Autodesk Fusion 360 part; units mm, degrees
(part 4 of 4)
sketch "Skizze66" plane through (0, 21.5, 0) normal (0, -1, 0) x (1, 0, 0)
  line L0 (56.5, -5) -> (51.5, -5)
  line L1 (51.5, -5) -> (51.5, -9.5)
  line L2 (51.5, -9.5) -> (31, -9.5)
  line L3 (31, -9.5) -> (31, -19.2)
  line L4 (31, -19.2) -> (32.5, -19.2)
  line L5 (32.5, -19.2) -> (32.5, -19)
  arc A0 (33.5, -18) -> (32.5, -19) centre (33.5, -19) ccw
  line L6 (33.5, -18) -> (38.5, -18)
  arc A1 (38.5, -18) -> (39.5, -17) centre (38.5, -17) ccw
  line L7 (39.5, -17) -> (39.5, -12)
  arc A2 (40.5, -11) -> (39.5, -12) centre (40.5, -12) ccw
  line L8 (40.5, -11) -> (56.5, -11)
  line L9 (56.5, -11) -> (56.5, -5)
  circle A3 centre (36, -14.5) radius 1.9
  line L10 (56.5, 5) -> (56.5, -5)
  line L11 (56.5, 5) -> (51.5, 5)
  line L12 (51.5, -5) -> (51.5, 5)
  line L13 (51.5, -5) -> (56.5, -5)
  circle A4 centre (-3.5, 16) radius 6.5
  line L14 (-21.5, -1.5) -> (-21.5, -23.5)
  line L15 (-21.5, -23.5) -> (5.5, -23.5)
  line L16 (5.5, -23.5) -> (5.5, -1.5)
  line L17 (5.5, -1.5) -> (-21.5, -1.5)
  line L18 (37.3325, 4.5) -> (48.5, 4.5)
  arc A5 (48.5, 4.5) -> (48.5, 7.5) centre (48.5, 6) ccw
  line L19 (48.5, 7.5) -> (37.3325, 7.5)
  arc A6 (37.3325, 7.5) -> (37.3325, 4.5) centre (37.3325, 6) ccw
  line L20 (12.5, 2.5057) -> (20.5, 2.5057)
  arc A7 (20.5, 2.5057) -> (20.5, 4.5057) centre (20.5, 3.5057) ccw
  line L21 (20.5, 4.5057) -> (12.5, 4.5057)
  arc A8 (12.5, 4.5057) -> (12.5, 2.5057) centre (12.5, 3.5057) ccw
  line L22 (12.5, -15.2086) -> (20.5, -15.2086)
  arc A9 (20.5, -15.2086) -> (20.5, -13.2086) centre (20.5, -14.2086) ccw
  line L23 (20.5, -13.2086) -> (12.5, -13.2086)
  arc A10 (12.5, -13.2086) -> (12.5, -15.2086) centre (12.5, -14.2086) ccw
  arc A11 (-34, 4.5) -> (-34, 7.5) centre (-34, 6) ccw
  line L24 (-34, 7.5) -> (-45, 7.5)
  arc A12 (-45, 7.5) -> (-45, 4.5) centre (-45, 6) ccw
  line L25 (-45, 4.5) -> (-34, 4.5)
  arc A13 (-34, -13.5) -> (-34, -10.5) centre (-34, -12) ccw
  line L26 (-34, -10.5) -> (-45, -10.5)
  arc A14 (-45, -10.5) -> (-45, -13.5) centre (-45, -12) ccw
  line L27 (-45, -13.5) -> (-34, -13.5)
  arc A15 (-34, 10.5) -> (-34, 13.5) centre (-34, 12) ccw
  line L28 (-34, 13.5) -> (-45, 13.5)
  arc A16 (-45, 13.5) -> (-45, 10.5) centre (-45, 12) ccw
  line L29 (-45, 10.5) -> (-34, 10.5)
  line L30 (12.5, -10.78) -> (20.5, -10.78)
  arc A17 (20.5, -10.78) -> (20.5, -8.78) centre (20.5, -9.78) ccw
  line L31 (20.5, -8.78) -> (12.5, -8.78)
  arc A18 (12.5, -8.78) -> (12.5, -10.78) centre (12.5, -9.78) ccw
  line L32 (20.5, 8.9343) -> (12.5, 8.9343)
  arc A19 (12.5, 8.9343) -> (12.5, 6.9343) centre (12.5, 7.9343) ccw
  line L33 (12.5, 6.9343) -> (20.5, 6.9343)
  arc A20 (20.5, 6.9343) -> (20.5, 8.9343) centre (20.5, 7.9343) ccw
  line L34 (37.3325, -1.5) -> (48.5, -1.5)
  arc A21 (48.5, -1.5) -> (48.5, 1.5) centre (48.5, 0) ccw
  line L35 (48.5, 1.5) -> (37.3325, 1.5)
  arc A22 (37.3325, 1.5) -> (37.3325, -1.5) centre (37.3325, 0) ccw
  arc A23 (20.5, -1.9228) -> (20.8852, 0) centre (20.5, -0.9228) ccw
  line L36 (20.8852, 0) -> (12.1148, 0)
  arc A24 (12.1148, 0) -> (12.5, -1.9228) centre (12.5, -0.9228) ccw
  line L37 (12.5, -1.9228) -> (20.5, -1.9228)
  line L38 (20.5, -22.0657) -> (20.5, -19.6371)
  arc A25 (20.5, -19.6371) -> (20.5, -17.6371) centre (20.5, -18.6371) ccw
  line L39 (20.5, -17.6371) -> (12.5, -17.6371)
  arc A26 (12.5, -17.6371) -> (12.5, -19.6371) centre (12.5, -18.6371) ccw
  line L40 (12.5, -19.6371) -> (12.5, -22.0657)
  arc A27 (12.5, -22.0657) -> (12.5, -24.0657) centre (12.5, -23.0657) ccw
  line L41 (12.5, -24.0657) -> (20.5, -24.0657)
  arc A28 (20.5, -24.0657) -> (20.5, -22.0657) centre (20.5, -23.0657) ccw
  line L42 (-34, 1.5) -> (-45, 1.5)
  arc A29 (-45, 1.5) -> (-45, -1.5) centre (-45, 0) ccw
  line L43 (-45, -1.5) -> (-34, -1.5)
  arc A30 (-34, -1.5) -> (-34, 1.5) centre (-34, 0) ccw
  arc A31 (-34, -7.5) -> (-34, -4.5) centre (-34, -6) ccw
  line L44 (-34, -4.5) -> (-45, -4.5)
  arc A32 (-45, -4.5) -> (-45, -7.5) centre (-45, -6) ccw
  line L45 (-45, -7.5) -> (-34, -7.5)
  line L46 (37.3325, -7.5) -> (48.5, -7.5)
  arc A33 (48.5, -7.5) -> (48.5, -4.5) centre (48.5, -6) ccw
  line L47 (48.5, -4.5) -> (37.3325, -4.5)
  arc A34 (37.3325, -4.5) -> (37.3325, -7.5) centre (37.3325, -6) ccw
  line L48 (-22.3, -10.5) -> (-30, -10.5)
  line L49 (-30, -10.5) -> (-30, -18.5)
  line L50 (-30, -18.5) -> (-22.3, -18.5)
  line L51 (-22.3, -18.5) -> (-22.3, -10.5)
  line L52 (36, 11) -> (56.5, 11)
  line L53 (56.5, 11) -> (56.5, -11)
  line L54 (56.5, -11) -> (36, -11)
  arc A35 (36, -11) -> (32.5, -14.5) centre (36, -14.5) ccw
  line L55 (32.5, -14.5) -> (32.5, -27.5)
  line L56 (32.5, -27.5) -> (-32, -27.5)
  line L57 (-32, -27.5) -> (-32, -25)
  arc A36 (-32, -25) -> (-36, -21) centre (-36, -25) ccw
  line L58 (-36, -21) -> (-43, -21)
  line L59 (-43, -21) -> (-57.5, -6.5)
  line L60 (-57.5, -6.5) -> (-57.5, 6.5)
  line L61 (-57.5, 6.5) -> (-43, 21)
  line L62 (-43, 21) -> (-36, 21)
  arc A37 (-36, 21) -> (-32, 25) centre (-36, 25) ccw
  line L63 (-32, 25) -> (-32, 27.5)
  line L64 (-32, 27.5) -> (10.5, 27.5)
  line L65 (10.5, 27.5) -> (10.5, 21.5)
  line L66 (10.5, 21.5) -> (12, 21.5)
  line L67 (12, 21.5) -> (12, 11.5)
  line L68 (12, 11.5) -> (21, 11.5)
  line L69 (21, 11.5) -> (21, 21.5)
  line L70 (21, 21.5) -> (22.5, 21.5)
  line L71 (22.5, 21.5) -> (22.5, 27.5)
  line L72 (22.5, 27.5) -> (32.5, 27.5)
  line L73 (32.5, 27.5) -> (32.5, 14.5)
  arc A38 (32.5, 14.5) -> (36, 11) centre (36, 14.5) ccw
  line L74 (20.5, -7.58) -> (20.5, -6.3514)
  arc A39 (20.5, -6.3514) -> (20.5, -4.3514) centre (20.5, -5.3514) ccw
  line L75 (20.5, -4.3514) -> (12.5, -4.3514)
  arc A40 (12.5, -4.3514) -> (12.5, -6.3514) centre (12.5, -5.3514) ccw
  line L76 (12.5, -6.3514) -> (12.5, -7.58)
  line L77 (12.5, -7.58) -> (20.5, -7.58)
  line L78 (51.5, 5) -> (56.5, 5)
  line L79 (56.5, 5) -> (56.5, 11)
  line L80 (56.5, 11) -> (40.5, 11)
  arc A41 (39.5, 12) -> (40.5, 11) centre (40.5, 12) ccw
  line L81 (39.5, 12) -> (39.5, 17)
  arc A42 (39.5, 17) -> (38.5, 18) centre (38.5, 17) ccw
  line L82 (38.5, 18) -> (33.5, 18)
  arc A43 (32.5, 19) -> (33.5, 18) centre (33.5, 19) ccw
  line L83 (32.5, 19) -> (32.5, 19.2)
  line L84 (32.5, 19.2) -> (31, 19.2)
  line L85 (31, 19.2) -> (31, 9.5)
  line L86 (31, 9.5) -> (51.5, 9.5)
  line L87 (51.5, 9.5) -> (51.5, 5)
  circle A44 centre (36, 14.5) radius 1.9
extrude "Extrusion72" cut sketch "Skizze66" against normal blind 3 contours L0 L1 L2 L3 L4 L5 L8 L9 L13 L53 L54 A35 L55 | L0 L10 L11 L12 L13 L53 L78 | L11 L52 L53 L73 A38 L78 L79 L80 L83 L84 L85 L86 L87 | A0 L6 A1 L7 A2 L54 A35 L55 | L52 L73 A38 A41 L81 A42 L82 A43 bodies 2
sketch "Skizze67" plane through (0, 16, 0) normal (0, -1, 0) x (1, 0, 0)
  circle A0 centre (-36, -25) radius 1.9
  line L0 (-18.0278, -27.5) -> (-18.0278, -26)
  line L1 (-18.0278, -26) -> (-23, -26)
  line L2 (-23, -26) -> (-31, -26)
  line L3 (-31, -26) -> (-31, -20)
  line L4 (-31, -20) -> (-41.8787, -20)
  line L5 (-41.8787, -20) -> (-51.5218, -10.3569)
  line L6 (-51.5218, -10.3569) -> (-51.5218, -5)
  line L7 (-51.5218, -5) -> (-57.5, -5)
  line L8 (-57.5, -5) -> (-57.5, -6.5)
  line L9 (-57.5, -6.5) -> (-42.5, -21.5)
  line L10 (-42.5, -21.5) -> (-38.922, -26.9266)
  arc A1 (-38.922, -26.9266) -> (-34.8649, -28.3108) centre (-36, -25) ccw
  line L11 (-34.8649, -28.3108) -> (-32.5, -27.5)
  line L12 (-32.5, -27.5) -> (-18.0278, -27.5)
  line L13 (-51.5218, 5) -> (-51.5218, -5)
  line L14 (-51.5218, 5) -> (-57.5, 5)
  line L15 (-57.5, -5) -> (-57.5, 5)
  line L16 (-57.5, -5) -> (-51.5218, -5)
  line L17 (-44.7071, 17.1716) -> (-47.5355, 14.3431)
  line L18 (-44.7071, 17.1716) -> (-45.7678, 18.2322)
  line L19 (-48.5962, 15.4038) -> (-45.7678, 18.2322)
  line L20 (-48.5962, 15.4038) -> (-47.5355, 14.3431)
extrude "Extrusion73" cut sketch "Skizze67" 3 faces at (-53.5145, 16, 7.2856) (-36.3402, 16, 21.0351) (24.5093, 16, -27) against normal blind 3 on bodies 2 bodies 2
extrude "Extrusion74" add 2 faces at (54.8333, 21.5, 8.5) (54.8333, 21.5, -8.5) along direction (0, 1, 0) blind 3 on bodies 1 bodies 1
extrude "Extrusion75" add 3 faces at (27.1759, 16, -27) (-53.5145, 16, 7.2856) (-53.5145, 16, -7.2856) along direction (0, 1, 0) blind 3 on bodies 1 bodies 1
sketch "Skizze68" plane through (0, 19, 0) normal (0, 1, 0) x (-1, 0, 0)
  line L0 (18.0278, -26) -> (18.0278, -27.5)
  line L1 (18.0278, -27.5) -> (32.5, -27.5)
  line L2 (32.5, -27.5) -> (33.8276, -28.3587)
  arc A0 (33.8276, -28.3587) -> (39.5022, -26.9326) centre (36, -25) ccw
  line L3 (39.5022, -26.9326) -> (42.5, -21.5)
  line L4 (42.5, -21.5) -> (57.5, -6.5)
  line L5 (57.5, -6.5) -> (57.5, -5)
  line L6 (57.5, -5) -> (51.5218, -5)
  line L7 (51.5218, -5) -> (51.5218, -10.3569)
  line L8 (51.5218, -10.3569) -> (41.8787, -20)
  line L9 (41.8787, -20) -> (31, -20)
  line L10 (31, -20) -> (31, -26)
  line L11 (31, -26) -> (18.0278, -26)
  circle A1 centre (36, -25) radius 1.9
  line L12 (51.5218, -5) -> (51.5218, 5)
  line L13 (51.5218, -5) -> (57.5, -5)
  line L14 (57.5, 5) -> (57.5, -5)
  line L15 (57.5, 5) -> (51.5218, 5)
  line L16 (-56.5, -5) -> (-56.5, 5)
  line L17 (-56.5, -5) -> (-51.5, -5)
  line L18 (-51.5, 5) -> (-51.5, -5)
  line L19 (-51.5, 5) -> (-56.5, 5)
  line L20 (-18.0278, -26) -> (0, -26)
  line L21 (-18.0278, -26) -> (-18.0278, -27.5)
  line L22 (18.0278, -27.5) -> (-18.0278, -27.5)
  line L23 (18.0278, -27.5) -> (18.0278, -26)
  line L24 (0, -26) -> (18.0278, -26)
extrude "Extrusion76" add sketch "Skizze68" against normal blind 17 contours L0 L20 L21 L22 L23 L24 | L6 L12 L13 L14 L15 bodies 1
sketch "Skizze69" plane through (0, 24.5, 0) normal (0, 1, 0) x (-1, 0, 0)
  circle A0 centre (-36, 14.5) radius 1.9
  arc A1 (-39.5, 18) -> (-40.5, 17) centre (-39.5, 17) ccw
  line L0 (-40.5, 17) -> (-40.5, 12)
  arc A2 (-41.5, 11) -> (-40.5, 12) centre (-41.5, 12) ccw
  line L1 (-41.5, 11) -> (-56.5, 11)
  line L2 (-56.5, 11) -> (-56.5, 5)
  line L3 (-56.5, 5) -> (-51.5, 5)
  line L4 (-51.5, 5) -> (-51.5, 9.5)
  line L5 (-51.5, 9.5) -> (-31, 9.5)
  line L6 (-31, 9.5) -> (-31, 19)
  line L7 (-31, 19) -> (-32.5, 19)
  arc A3 (-33.5, 18) -> (-32.5, 19) centre (-33.5, 19) ccw
  line L8 (-33.5, 18) -> (-39.5, 18)
  line L9 (-56.5, -5) -> (-56.5, 5)
  line L10 (-56.5, -5) -> (-51.5, -5)
  line L11 (-51.5, 5) -> (-51.5, -5)
  line L12 (-51.5, 5) -> (-56.5, 5)
extrude "Extrusion77" add sketch "Skizze69" against normal blind 10 contours L3 L9 L10 L11 L12 bodies 1
sketch "Skizze70" plane through (0, 0, -27.5) normal (0, 0, -1) x (-1, 0, 0)
  line L0 (-13, 2) -> (-13, 0)
  line L1 (-13, 0) -> (13, 0)
  line L2 (13, 0) -> (13, 2)
  line L3 (13, 2) -> (20.1, 2)
  line L4 (20.1, 2) -> (20.1, 9)
  line L5 (20.1, 9) -> (22, 9)
  line L6 (22, 9) -> (22, 0)
  line L7 (22, 0) -> (32.5, 0)
  line L8 (32.5, 0) -> (32.5, 19)
  line L9 (32.5, 19) -> (-32.5, 19)
  line L10 (-32.5, 19) -> (-32.5, 0)
  line L11 (-32.5, 0) -> (-22, 0)
  line L12 (-22, 0) -> (-22, 9)
  line L13 (-22, 9) -> (-20.1, 9)
  line L14 (-20.1, 9) -> (-20.1, 2)
  line L15 (-20.1, 2) -> (-13, 2)
  arc A0 (18.7617, 19) -> (-18.7617, 19) centre (0, 22) ccw
  circle A1 centre (0, 22) radius 19
extrude "Extrusion78" cut sketch "Skizze70" against normal blind 1.5 contours L9 A1 bodies 1
sketch "Skizze71" plane through (-57.5, 0, 0) normal (-1, 0, 0) x (0, 0, 1)
  line L0 (6.5, 19) -> (-6.5, 19)
  line L1 (-6.5, 19) -> (-6.5, 0)
  line L2 (-6.5, 0) -> (6.5, 0)
  line L3 (6.5, 0) -> (6.5, 19)
  circle A0 centre (0, 19) radius 4
  dimension "d349" = 8
  measures "d349" diameter of A0
extrude "Extrusion79" cut sketch "Skizze71" against normal blind 6 contours L0 A0 | L0 A0 bodies 1 2
sketch "Skizze72" plane through (56.5, 0, 0) normal (1, 0, 0) x (0, 0, -1)
  line L0 (11, 24.5) -> (-11, 24.5)
  line L1 (-11, 24.5) -> (-11, 0)
  line L2 (-11, 0) -> (11, 0)
  line L3 (11, 0) -> (11, 24.5)
  circle A0 centre (0, 24.5) radius 4.5
  dimension "d352" = 9
  measures "d352" diameter of A0
extrude "Extrusion80" cut sketch "Skizze72" against normal blind 5.5 contours L0 A0 | L0 A0 bodies 1 2
sketch "Skizze73" plane through (-32, 0, 32) normal (-0.707107, 0, 0.707107) x (0.707107, 0, 0.707107)
  line L0 (-19.7385, 19) -> (-14.8492, 19)
  line L1 (-14.8492, 19) -> (-14.8492, 33.5)
  line L2 (-14.8492, 33.5) -> (-15.5563, 33.5)
  line L3 (-15.5563, 33.5) -> (-15.5563, 47)
  line L4 (-15.5563, 47) -> (-36.0624, 47)
  line L5 (-36.0624, 47) -> (-36.0624, 19)
  line L6 (-36.0624, 19) -> (-23.2026, 19)
  arc A0 (-19.7385, 19) -> (-23.2026, 19) centre (-21.4706, 18) ccw
  line L7 (-23.2026, 19) -> (-19.7385, 19)
extrude "Extrusion81" add sketch "Skizze73" against normal blind 1.5 contours A0 L7 bodies 2
sketch "Skizze74" plane through (-32, 0, 32) normal (-0.707107, 0, 0.707107) x (0.707107, 0, 0.707107)
  line L0 (-36.0624, 19) -> (-14.8492, 19)
  line L1 (-14.8492, 19) -> (-14.8492, 33.5)
  line L2 (-14.8492, 33.5) -> (-15.5563, 33.5)
  line L3 (-15.5563, 33.5) -> (-15.5563, 47)
  line L4 (-15.5563, 47) -> (-36.0624, 47)
  line L5 (-36.0624, 47) -> (-36.0624, 19)
  circle A0 centre (-20.8492, 20.5) radius 1.5
  line L6 (-15.4706, 19) -> (-29.108, 19)
  line L7 (-19.3492, 20.5) -> (-19.3492, 19)
  line L8 (-22.3492, 20.5) -> (-22.3492, 19)
  dimension "d359" = 3
  dimension "d360" = 6
  measures "d359" diameter of A0
  measures "d360" distance of L1 origin
extrude "Extrusion82" cut sketch "Skizze74" against normal blind 1.5 contours L0 A0 L6 L8 | L0 A0 L6 L7 | A0 bodies 2
extrude "Extrusion83" add 4 faces at (-28.65, 10, -25.2151) (27.0473, 10, -25.2982) (28.65, 10, 25.2151) (-28.65, 10, 25.2151) along direction (0, 1, 0) blind 3 on bodies 1 bodies 1
extrude "Extrusion84" add 2 faces at (16, 44, -31.5333) (-16, 44, -35.5667) along direction (0, 1, 0) blind 3 on bodies 2 bodies 2
extrude "Extrusion85" cut 2 faces at (15.3333, 42, -34.5667) (-17.7, 42, -31.0333) along direction (0, 1, 0) blind 0.2 on bodies 2 bodies 2
sketch "Skizze75" plane through (0, 0, -39.6) normal (0, 0, -1) x (-1, 0, 0)
  line L0 (-22, 47) -> (-22, 35.2606)
  line L1 (-22, 35.2606) -> (-20, 35.2606)
  line L2 (-20, 35.2606) -> (-13, 42)
  line L3 (-13, 42) -> (-13, 47)
  line L4 (-13, 47) -> (-22, 47)
  line L5 (-13, 42.2) -> (-20, 35.2606)
  line L6 (13, 42.2) -> (20, 35)
  line L7 (13, 42) -> (20, 35)
  line L8 (20, 35) -> (22, 35)
  line L9 (22, 35) -> (22, 47)
  line L10 (22, 47) -> (13, 47)
  line L11 (13, 47) -> (13, 42)
extrude "Extrusion86" cut sketch "Skizze75" against normal blind 1.5 contours L2 L3 L5 | L6 L7 L11 bodies 2
extrude "Extrusion87" cut 4 faces at (39.6333, 33.5, 14.5) (39.6333, 33.5, -14.5) (-39.9603, 33.5, -24.3831) (-39.9603, 33.5, 24.3831) along direction (0, -1, 0) blind 3 on bodies 2 bodies 2
sketch "Skizze76" plane through (-32, 0, -32) normal (-0.707107, 0, -0.707107) x (-0.707107, 0, 0.707107)
  line L0 (15.5563, 47) -> (15.5563, 30.5)
  line L1 (15.5563, 30.5) -> (14.8492, 30.5)
  line L2 (14.8492, 30.5) -> (14.8492, 19)
  line L3 (14.8492, 19) -> (36.0624, 19)
  line L4 (36.0624, 19) -> (36.0624, 47)
  line L5 (36.0624, 47) -> (15.5563, 47)
  circle A0 centre (20.8492, 20.5) radius 1.5
  line L6 (22.3492, 20.5) -> (22.3492, 18.9)
  line L7 (19.3492, 20.5) -> (19.3492, 18.9)
  line L8 (14.8492, 19) -> (36.0624, 19)
  dimension "d373" = 3
  dimension "d374" = 6
  measures "d373" diameter of A0
  measures "d374" distance of L2 origin
extrude "Extrusion88" cut sketch "Skizze76" against normal blind 1.5 contours L3 A0 L6 L8 | L3 A0 L7 L8 | A0 bodies 2
extrude "Extrusion89" add 6 faces at (16, 45, -39.6) (18.3333, 40.4869, -39.6) (-19, 45, -39.6) (-18.3333, 40.4, -39.6) (18.3333, 3.6667, -39.6) (-18.3333, 3.6667, -39.6) along direction (0, 0, -1) blind 1 on bodies 1 2 bodies 2 1
extrude "Extrusion90" cut 7 faces at (17.7339, 39.7535, -38.1) (15.4006, 42.1333, -38.1) (17.7, 4.3333, -38.1) (-17.7, 4.3333, -38.1) (-20.0333, 37.3333, -38.1) (-15.4315, 42.1333, -38.1) (-17.7315, 39.6667, -38.1) along direction (0, 0, -1) blind 1 on bodies 1 2 bodies 1 2
equation "d18 = d17"
equation "d19 = d17"
equation "d20 = d17"
equation "d24 = d23"
equation "d25 = d23"
equation "d26 = d23"
equation "d42 = d41"
equation "d43 = d41"
equation "d44 = d41"
equation "d45 = d41"
equation "d46 = d41"
equation "d47 = d41"
equation "d48 = d41"
equation "d49 = d41"
equation "d50 = d41"
equation "d51 = d41"
equation "d52 = d41"
equation "d53 = d41"
equation "d54 = d41"
equation "d98 = d95 / 2"
equation "d99 = d96 / 2"
equation "d198 = d197"
equation "d199 = d197"
equation "d200 = d197"
equation "d229 = d224 / 2"
equation "d230 = d225 / 2"
equation "d231 = ( d225 - 32 mm ) / 2"
equation "d232 = d231"
equation "d233 = d228"
equation "d234 = d231"
equation "d235 = d231"
named bodies: "Case_bottom", "Case_top", "Rotary_Knob"
